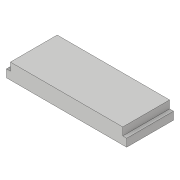
# Autodesk Inventor part: Lidar Sensor Case Piece 3
Saved by Autodesk Inventor 2018.3 (Build 223284000, 284)
## iProperties
Created: 2019-02-26
Part Number: Lidar Sensor Case Piece 3
Material: Generic
Document SubType Name: Modeling
Designer: aye06091
Mass: 5.72267 g
Surface Area: 27.0564 cm^2
Volume: 5.72267 cm^3
Density: 1 g/cm^3
Appearance: Default
Author: aye06091
Autodesk Inventor part; units mm, degrees
ref_plane "YZ Plane" through (0, 0, 0) normal (1, 0, 0) x (0, 1, 0)
ref_plane "XZ Plane" through (0, 0, 0) normal (0, 1, 0) x (-1, 0, 0)
ref_plane "XY Plane" through (0, 0, 0) normal (0, 0, 1) x (1, 0, 0)
sketch "Sketch1" plane through (0, 0, 0) normal (0, 1, 0) x (-1, 0, 0)
  line L0 (0, 0) -> (-48.895, 0)
  line L1 (-48.895, 0) -> (-48.895, 19.05)
  line L2 (-48.895, 19.05) -> (0, 19.05)
  line L3 (0, 19.05) -> (0, 0)
  dimension "d0" = 48.895
  dimension "d1" = 19.05
  constraints: 8 end point, 2 parallel, 1 horizontal, 1 perpendicular
  measures "d0" distance of L0.start L0.end
  measures "d1" distance of L2.end L0.start
extrude "Extrusion1" add sketch "Sketch1" along normal blind 6.35
sketch "Sketch5" plane through (0, 6.35, 0) normal (0, 1, 0) x (1, 0, 0)
  line L0 (0, 0) -> (0, -19.05) projected
  line L1 (0, -19.05) -> (48.895, -19.05) projected
  line L2 (48.895, -19.05) -> (48.895, 0) projected
  line L3 (0, 0) -> (1.5875, 0)
  line L4 (1.5875, 0) -> (1.5875, -19.05)
  line L5 (1.5875, -19.05) -> (0, -19.05)
  line L6 (0, -19.05) -> (0, 0)
  line L7 (48.895, 0) -> (47.3075, 0)
  line L8 (47.3075, 0) -> (47.3075, -19.05)
  line L9 (47.3075, -19.05) -> (48.895, -19.05)
  line L10 (48.895, -19.05) -> (48.895, 0)
  dimension "d17" = 1.5875
  dimension "d18" = 1.5875
  constraints: 16 end point, 4 parallel, 2 horizontal, 2 perpendicular, 2 point on line
  measures "d17" distance between parallel lines of L0 L4
  measures "d18" distance between parallel lines of L8 L2
extrude "Extrusion5" cut sketch "Sketch5" against normal blind 3.175
body "Solid1"
